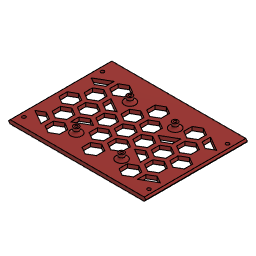
MCU Tray - BTT SKR Pico (Autodesk Fusion 360 design; units mm, degrees)
Autodesk Fusion 360 part; units mm, degrees
sketch "Sketch1" plane through (0, 0, 0) normal (0, 1, 0) x (1, 0, 0)
  line L0 (72.5, 2) -> (-72.5, 2)
  line L1 (-72.5, 2) -> (-72.5, -2) construction
  line L2 (-72.5, -2) -> (72.5, -2)
  line L3 (72.5, -2) -> (72.5, 2) construction
  line L4 (72.5, 2) -> (-72.5, -2) construction
  line L5 (-72.5, 2) -> (72.5, -2) construction
  line L6 (-72.5, 0) -> (-74.3, 0) construction
  line L7 (-72.5, -2) -> (-74.3, -0.2)
  line L8 (-74.3, 0.2) -> (-72.5, 2)
  line L9 (-74.3, -0.2) -> (-74.3, 0)
  line L10 (-74.3, 0) -> (-74.3, 0.2)
  line L11 (0, 0) -> (0, -2) construction
  line L12 (72.5, -2) -> (74.3, -0.2)
  line L13 (74.3, -0.2) -> (74.3, 0)
  line L14 (74.3, 0) -> (74.3, 0.2)
  line L15 (74.3, 0.2) -> (72.5, 2)
  dimension "d1" = 145
  dimension "d2" = 4
  dimension "d3" = 0.2
  constraint horizontal L0
  constraint perpendicular L0 L1
  constraint parallel L0 L2
  constraint parallel L1 L3
  constraint coincident L4 L11.start
  constraint coincident L5 L11.start
  constraint coincident L11.start origin
  constraint midpoint L1 L6.start
  constraint perpendicular L1 L6
  constraint coincident L5 L0.end
  constraint coincident L0 L1.start
  constraint perpendicular L6 L9
  constraint perpendicular L6 L10
  constraint midpoint L2 L11.end
  constraint symmetric L1.end L11 L2.end
  constraint symmetric L0.end L11 L0.start
  constraint symmetric L7.end L11 L12.end
  constraint symmetric L6.end L11 L13.end
  constraint symmetric L8.start L11 L14.end
  measures "d1" distance of L1.end L2.end
  measures "d2" distance of L0.end L1.end
  measures "d3" distance of L7.end L6.end
extrude "Extrude1" add sketch "Sketch1" along normal blind 190 and the other way blind 15
sketch "Sketch2" plane through (0, 0, 2) normal (0, 0, 1) x (-1, 0, 0)
  line L0 (72.5, 15) -> (-72.5, 15)
  line L1 (-72.5, 15) -> (-72.5, -190)
  line L2 (-72.5, -190) -> (72.5, -190)
  line L3 (72.5, -190) -> (72.5, 15)
  line L4 (0, 0) -> (0, -13.083) construction
  circle A0 centre (-67.6414, -9.9998) radius 2.3
  line L5 (72.6414, -59.8458) -> (72.6414, 0.0002) construction
  circle A1 centre (67.6414, -9.9998) radius 2.3
  line L6 (72.5, -190) -> (72.5, 15)
  line L7 (72.6414, 0.0002) -> (67.6414, 0.0002) construction
  line L8 (67.6414, 0.0002) -> (67.6414, -9.9998) construction
  line L9 (67.6414, -9.9998) -> (72.6414, -9.9998) construction
  line L10 (72.6414, -9.9998) -> (72.6414, 0.0002) construction
  line L11 (67.6414, -9.9998) -> (67.6414, -94.9998) construction
  circle A2 centre (67.6414, -94.9998) radius 2.3
  circle A3 centre (-67.6414, -94.9998) radius 2.3
  circle A4 centre (-67.6414, -9.9998) radius 1.8
  circle A5 centre (67.6414, -9.9998) radius 1.8
  circle A6 centre (67.6414, -94.9998) radius 1.8
  circle A7 centre (-67.6414, -94.9998) radius 1.8
  dimension "d14" = 5
  dimension "d15" = 10
  dimension "d16" = 4.6
  dimension "d17" = 85
  dimension "d18" = 4.6
  dimension "d59" = 3.6
  dimension "d60" = 3.6
  dimension "d61" = 3.6
  dimension "d62" = 3.6
  constraint coincident L4.start origin
  constraint vertical L4
  constraint symmetric L4 A0 A1
  constraint horizontal L7
  constraint vertical L8
  constraint horizontal L9
  constraint vertical L10
  constraint coincident A1.centre L8.end
  constraint perpendicular L9 L11
  constraint coincident L11.end A2.centre
  constraint symmetric L4 A2 A3
  constraint concentric A0 A4
  constraint concentric A1 A5
  constraint concentric A2 A6
  constraint concentric A3 A7
  measures "d14" distance of L5.end L7.end
  measures "d15" distance of L5.end L9.end
  measures "d16" diameter of A1
  measures "d17" distance of A1.centre L11.end
  measures "d18" diameter of A2
  measures "d59" diameter of A4
  measures "d60" diameter of A5
  measures "d61" diameter of A6
  measures "d62" diameter of A7
extrude "Extrude2" cut sketch "Sketch2" against normal up to surface (4 mm away) contours A0 | A1 | A2 | A3 | A4 | A5 | A6 | A7
extrude "Extrude3" cut 1 faces at (24.1667, 190, 0.6667) along direction (0, -1, 0) blind 40.154
extrude "Extrude10" add sketch "Sketch2" against normal blind 4 contours A0 | A1 | A2 | A3
sketch "Sketch3" plane through (0, 0, 2) normal (0, 0, 1) x (-1, 0, 0)
  line L0 (-72.5, -149.846) -> (72.5, -149.846)
  line L1 (72.5, -149.846) -> (72.5, 15)
  line L2 (72.5, 15) -> (-72.5, 15)
  line L3 (-72.5, 15) -> (-72.5, -149.846)
  line L4 (67.6414, -94.9998) -> (-67.6414, -9.9998) construction
  line L5 (-24.5, -23.4998) -> (24.5, -81.4998) construction
  line L6 (24.5, -23.4998) -> (-24.5, -81.4998) construction
  circle A0 centre (24.5, -81.4998) radius 2.35
  circle A1 centre (-24.5, -81.4998) radius 3
  circle A2 centre (24.5, -81.4998) radius 3
  circle A3 centre (-24.5, -81.4998) radius 2.35
  circle A4 centre (24.5, -23.4998) radius 2.35
  circle A5 centre (24.5, -23.4998) radius 3
  circle A6 centre (-24.5, -23.4998) radius 3
  circle A7 centre (-24.5, -23.4998) radius 2.35
  circle A8 centre (24.5, -23.4998) radius 1.4
  circle A9 centre (-24.5, -23.4998) radius 1.4
  circle A10 centre (-24.5, -81.4998) radius 1.4
  circle A11 centre (24.5, -81.4998) radius 1.4
  circle A12 centre (67.6414, -94.9998) radius 1.8
  circle A13 centre (-67.6414, -94.9998) radius 1.8
  circle A14 centre (67.6414, -9.9998) radius 1.8
  circle A15 centre (-67.6414, -9.9998) radius 1.8
  point P0 (0, -52.4998)
  dimension "d19" = 49
  dimension "d20" = 58
  dimension "d21" = 4.7
  dimension "d22" = 6
  dimension "d23" = 6
  dimension "d24" = 4.7
  dimension "d25" = 4.7
  dimension "d26" = 6
  dimension "d27" = 6
  dimension "d28" = 4.7
  dimension "d33" = 2.8
  dimension "d34" = 2.8
  dimension "d35" = 2.8
  dimension "d36" = 2.8
  constraint coincident L5 P0
  constraint coincident L6 P0
  constraint midpoint L4 P0
  constraint coincident L5.end A0.centre
  constraint coincident L6.end A1.centre
  constraint concentric A0 A2
  constraint concentric A1 A3
  constraint coincident L6.start A4.centre
  constraint concentric A4 A5
  constraint coincident L5.start A6.centre
  constraint concentric A6 A7
  constraint concentric A4 A8
  constraint concentric A6 A9
  constraint concentric A1 A10
  measures "d19" distance of L5.end L6.end
  measures "d20" distance of L6.start L5.end
  measures "d21" diameter of A0
  measures "d22" diameter of A1
  measures "d23" diameter of A2
  measures "d24" diameter of A3
  measures "d25" diameter of A4
  measures "d26" diameter of A5
  measures "d27" diameter of A6
  measures "d28" diameter of A7
  measures "d33" diameter of A8
  measures "d34" diameter of A9
  measures "d35" diameter of A10
  measures "d36" diameter of A11
extrude "Extrude4" cut sketch "Sketch3" against normal blind 4 contours A8 | A9 | A10 | A11
extrude "Extrude5" add sketch "Sketch3" along normal blind 6 contours A0 | A1 | A2 | A3 | A4 | A5 | A6 | A7
extrude "Extrude7" cut 1 faces at (24.1667, -15, 0.6667) along direction (0, 1, 0) blind 15
extrude "Extrude8" cut 1 faces at (24.1667, 149.846, 0.6667) along direction (0, -1, 0) blind 40
sketch "Sketch4" plane through (0, 0, 2) normal (0, 0, 1) x (-1, 0, 0)
  line L0 (-72.5, -109.846) -> (72.5, -109.846)
  line L1 (72.5, -109.846) -> (72.5, 0)
  line L2 (72.5, 0) -> (-72.5, 0)
  line L3 (-72.5, 0) -> (-72.5, -109.846)
  line L4 (-24.5, -23.4998) -> (24.5, -81.4998) construction
  line L5 (24.5, -81.4998) -> (24.5, -23.4998) construction
  line L6 (24.5, -23.4998) -> (-24.5, -81.4998) construction
  line L7 (0, -43.4998) -> (-7.7942, -47.9998)
  line L8 (-7.7942, -47.9998) -> (-7.7942, -56.9998)
  line L9 (-7.7942, -56.9998) -> (0, -61.4998)
  line L10 (0, -61.4998) -> (7.7942, -56.9998)
  line L11 (7.7942, -56.9998) -> (7.7942, -47.9998)
  line L12 (7.7942, -47.9998) -> (0, -43.4998)
  line L13 (52.2058, -47.9998) -> (52.2058, -56.9998)
  line L14 (52.2058, -56.9998) -> (60, -61.4998)
  line L15 (60, -61.4998) -> (67.7942, -56.9998)
  line L16 (67.7942, -56.9998) -> (67.7942, -47.9998)
  line L17 (67.7942, -47.9998) -> (60, -43.4998)
  line L18 (60, -43.4998) -> (52.2058, -47.9998)
  line L19 (32.2058, -47.9998) -> (32.2058, -56.9998)
  line L20 (32.2058, -56.9998) -> (40, -61.4998)
  line L21 (40, -61.4998) -> (47.7942, -56.9998)
  line L22 (47.7942, -56.9998) -> (47.7942, -47.9998)
  line L23 (47.7942, -47.9998) -> (40, -43.4998)
  line L24 (40, -43.4998) -> (32.2058, -47.9998)
  line L25 (12.2058, -47.9998) -> (12.2058, -56.9998)
  line L26 (12.2058, -56.9998) -> (20, -61.4998)
  line L27 (20, -61.4998) -> (27.7942, -56.9998)
  line L28 (27.7942, -56.9998) -> (27.7942, -47.9998)
  line L29 (27.7942, -47.9998) -> (20, -43.4998)
  line L30 (20, -43.4998) -> (12.2058, -47.9998)
  line L31 (-27.7942, -47.9998) -> (-27.7942, -56.9998)
  line L32 (-27.7942, -56.9998) -> (-20, -61.4998)
  line L33 (-20, -61.4998) -> (-12.2058, -56.9998)
  line L34 (-12.2058, -56.9998) -> (-12.2058, -47.9998)
  line L35 (-12.2058, -47.9998) -> (-20, -43.4998)
  line L36 (-20, -43.4998) -> (-27.7942, -47.9998)
  line L37 (-47.7942, -47.9998) -> (-47.7942, -56.9998)
  line L38 (-47.7942, -56.9998) -> (-40, -61.4998)
  line L39 (-40, -61.4998) -> (-32.2058, -56.9998)
  line L40 (-32.2058, -56.9998) -> (-32.2058, -47.9998)
  line L41 (-32.2058, -47.9998) -> (-40, -43.4998)
  line L42 (-40, -43.4998) -> (-47.7942, -47.9998)
  line L43 (10, -60.8203) -> (2.2058, -65.3203)
  line L44 (2.2058, -65.3203) -> (2.2058, -74.3203)
  line L45 (2.2058, -74.3203) -> (10, -78.8203)
  line L46 (10, -78.8203) -> (17.7942, -74.3203)
  line L47 (17.7942, -74.3203) -> (17.7942, -65.3203)
  line L48 (17.7942, -65.3203) -> (10, -60.8203)
  line L49 (77.7942, -65.3203) -> (70, -60.8203) construction
  line L50 (70, -60.8203) -> (62.2058, -65.3203) construction
  line L51 (62.2058, -65.3203) -> (62.2058, -74.3203) construction
  line L52 (62.2058, -74.3203) -> (70, -78.8203) construction
  line L53 (77.7942, -74.3203) -> (77.7942, -65.3203) construction
  line L54 (70, -78.8203) -> (77.7942, -74.3203) construction
  line L55 (57.7942, -65.3203) -> (50, -60.8203)
  line L56 (50, -60.8203) -> (42.2058, -65.3203)
  line L57 (42.2058, -65.3203) -> (42.2058, -74.3203)
  line L58 (42.2058, -74.3203) -> (50, -78.8203)
  line L59 (57.7942, -74.3203) -> (57.7942, -65.3203)
  line L60 (50, -78.8203) -> (57.7942, -74.3203)
  line L61 (37.7942, -65.3203) -> (30, -60.8203)
  line L62 (30, -60.8203) -> (22.2058, -65.3203)
  line L63 (22.2058, -65.3203) -> (22.2058, -74.3203) construction
  line L64 (22.2058, -74.3203) -> (30, -78.8203) construction
  line L65 (37.7942, -74.3203) -> (37.7942, -65.3203)
  line L66 (30, -78.8203) -> (37.7942, -74.3203) construction
  line L67 (-2.2058, -65.3203) -> (-10, -60.8203)
  line L68 (-10, -60.8203) -> (-17.7942, -65.3203)
  line L69 (-17.7942, -65.3203) -> (-17.7942, -74.3203)
  line L70 (-17.7942, -74.3203) -> (-10, -78.8203)
  line L71 (-2.2058, -74.3203) -> (-2.2058, -65.3203)
  line L72 (-10, -78.8203) -> (-2.2058, -74.3203)
  line L73 (-22.2058, -65.3203) -> (-30, -60.8203)
  line L74 (-30, -60.8203) -> (-37.7942, -65.3203)
  line L75 (-37.7942, -65.3203) -> (-37.7942, -74.3203)
  line L76 (-37.7942, -74.3203) -> (-30, -78.8203) construction
  line L77 (-22.2058, -74.3203) -> (-22.2058, -65.3203) construction
  line L78 (-30, -78.8203) -> (-22.2058, -74.3203) construction
  line L79 (-67.7942, -47.9998) -> (-67.7942, -56.9998)
  line L80 (-67.7942, -56.9998) -> (-60, -61.4998)
  line L81 (-60, -61.4998) -> (-52.2058, -56.9998)
  line L82 (-52.2058, -56.9998) -> (-52.2058, -47.9998)
  line L83 (-52.2058, -47.9998) -> (-60, -43.4998)
  line L84 (-60, -43.4998) -> (-67.7942, -47.9998)
  line L85 (-42.2058, -65.3203) -> (-50, -60.8203)
  line L86 (-50, -60.8203) -> (-57.7942, -65.3203)
  line L87 (-57.7942, -65.3203) -> (-57.7942, -74.3203)
  line L88 (-57.7942, -74.3203) -> (-50, -78.8203)
  line L89 (-42.2058, -74.3203) -> (-42.2058, -65.3203)
  line L90 (-50, -78.8203) -> (-42.2058, -74.3203)
  line L91 (2.2058, -39.6793) -> (10, -44.1793)
  line L92 (10, -44.1793) -> (17.7942, -39.6793)
  line L93 (17.7942, -39.6793) -> (17.7942, -30.6793)
  line L94 (17.7942, -30.6793) -> (10, -26.1793)
  line L95 (10, -26.1793) -> (2.2058, -30.6793)
  line L96 (2.2058, -30.6793) -> (2.2058, -39.6793)
  line L97 (77.7942, -39.6793) -> (77.7942, -30.6793) construction
  line L98 (77.7942, -30.6793) -> (70, -26.1793) construction
  line L99 (70, -26.1793) -> (62.2058, -30.6793) construction
  line L100 (62.2058, -30.6793) -> (62.2058, -39.6793) construction
  line L101 (70, -44.1793) -> (77.7942, -39.6793) construction
  line L102 (62.2058, -39.6793) -> (70, -44.1793) construction
  line L103 (57.7942, -39.6793) -> (57.7942, -30.6793)
  line L104 (57.7942, -30.6793) -> (50, -26.1793)
  line L105 (50, -26.1793) -> (42.2058, -30.6793)
  line L106 (42.2058, -30.6793) -> (42.2058, -39.6793)
  line L107 (50, -44.1793) -> (57.7942, -39.6793)
  line L108 (42.2058, -39.6793) -> (50, -44.1793)
  line L109 (37.7942, -39.6793) -> (37.7942, -30.6793)
  line L110 (37.7942, -30.6793) -> (30, -26.1793) construction
  line L111 (30, -26.1793) -> (22.2058, -30.6793) construction
  line L112 (22.2058, -30.6793) -> (22.2058, -39.6793) construction
  line L113 (30, -44.1793) -> (37.7942, -39.6793)
  line L114 (22.2058, -39.6793) -> (30, -44.1793)
  line L115 (-2.2058, -39.6793) -> (-2.2058, -30.6793)
  line L116 (-2.2058, -30.6793) -> (-10, -26.1793)
  line L117 (-10, -26.1793) -> (-17.7942, -30.6793)
  line L118 (-17.7942, -30.6793) -> (-17.7942, -39.6793)
  line L119 (-10, -44.1793) -> (-2.2058, -39.6793)
  line L120 (-17.7942, -39.6793) -> (-10, -44.1793)
  line L121 (-22.2058, -39.6793) -> (-22.2058, -30.6793) construction
  line L122 (-22.2058, -30.6793) -> (-30, -26.1793) construction
  line L123 (-30, -26.1793) -> (-37.7942, -30.6793) construction
  line L124 (-37.7942, -30.6793) -> (-37.7942, -39.6793)
  line L125 (-30, -44.1793) -> (-22.2058, -39.6793)
  line L126 (-37.7942, -39.6793) -> (-30, -44.1793)
  line L127 (-42.2058, -39.6793) -> (-42.2058, -30.6793)
  line L128 (-42.2058, -30.6793) -> (-50, -26.1793)
  line L129 (-50, -26.1793) -> (-57.7942, -30.6793)
  line L130 (-57.7942, -30.6793) -> (-57.7942, -39.6793)
  line L131 (-50, -44.1793) -> (-42.2058, -39.6793)
  line L132 (-57.7942, -39.6793) -> (-50, -44.1793)
  line L133 (-87.7942, -47.9998) -> (-87.7942, -56.9998) construction
  line L134 (-87.7942, -56.9998) -> (-80, -61.4998) construction
  line L135 (-80, -61.4998) -> (-72.2058, -56.9998) construction
  line L136 (-72.2058, -56.9998) -> (-72.2058, -47.9998) construction
  line L137 (-72.2058, -47.9998) -> (-80, -43.4998) construction
  line L138 (-80, -43.4998) -> (-87.7942, -47.9998) construction
  line L139 (-62.2058, -65.3203) -> (-70, -60.8203) construction
  line L140 (-70, -60.8203) -> (-77.7942, -65.3203) construction
  line L141 (-77.7942, -65.3203) -> (-77.7942, -74.3203) construction
  line L142 (-77.7942, -74.3203) -> (-70, -78.8203) construction
  line L143 (-62.2058, -74.3203) -> (-62.2058, -65.3203) construction
  line L144 (-70, -78.8203) -> (-62.2058, -74.3203) construction
  line L145 (-62.2058, -39.6793) -> (-62.2058, -30.6793) construction
  line L146 (-62.2058, -30.6793) -> (-70, -26.1793) construction
  line L147 (-70, -26.1793) -> (-77.7942, -30.6793) construction
  line L148 (-77.7942, -30.6793) -> (-77.7942, -39.6793) construction
  line L149 (-70, -44.1793) -> (-62.2058, -39.6793) construction
  line L150 (-77.7942, -39.6793) -> (-70, -44.1793) construction
  line L151 (-67.7942, -82.9998) -> (-67.7942, -91.9998) construction
  line L152 (-67.7942, -91.9998) -> (-60, -96.4998) construction
  line L153 (-60, -96.4998) -> (-52.2058, -91.9998) construction
  line L154 (-52.2058, -91.9998) -> (-52.2058, -82.9998)
  line L155 (-52.2058, -82.9998) -> (-60, -78.4998)
  line L156 (-60, -78.4998) -> (-67.7942, -82.9998)
  line L157 (-47.7942, -91.9998) -> (-40, -96.4998)
  line L158 (-40, -96.4998) -> (-32.2058, -91.9998)
  line L159 (-32.2058, -91.9998) -> (-32.2058, -82.9998)
  line L160 (-32.2058, -82.9998) -> (-40, -78.4998)
  line L161 (-47.7942, -82.9998) -> (-47.7942, -91.9998)
  line L162 (-40, -78.4998) -> (-47.7942, -82.9998)
  line L163 (-27.7942, -91.9998) -> (-20, -96.4998)
  line L164 (-20, -96.4998) -> (-12.2058, -91.9998)
  line L165 (-12.2058, -91.9998) -> (-12.2058, -82.9998)
  line L166 (-12.2058, -82.9998) -> (-20, -78.4998)
  line L167 (-27.7942, -82.9998) -> (-27.7942, -91.9998)
  line L168 (-20, -78.4998) -> (-27.7942, -82.9998)
  line L169 (-7.7942, -91.9998) -> (0, -96.4998)
  line L170 (0, -96.4998) -> (7.7942, -91.9998)
  line L171 (7.7942, -91.9998) -> (7.7942, -82.9998)
  line L172 (7.7942, -82.9998) -> (0, -78.4998)
  line L173 (-7.7942, -82.9998) -> (-7.7942, -91.9998)
  line L174 (0, -78.4998) -> (-7.7942, -82.9998)
  line L175 (12.2058, -91.9998) -> (20, -96.4998)
  line L176 (20, -96.4998) -> (27.7942, -91.9998)
  line L177 (27.7942, -91.9998) -> (27.7942, -82.9998)
  line L178 (27.7942, -82.9998) -> (20, -78.4998)
  line L179 (12.2058, -82.9998) -> (12.2058, -91.9998)
  line L180 (20, -78.4998) -> (12.2058, -82.9998)
  line L181 (32.2058, -91.9998) -> (40, -96.4998)
  line L182 (40, -96.4998) -> (47.7942, -91.9998)
  line L183 (47.7942, -91.9998) -> (47.7942, -82.9998)
  line L184 (47.7942, -82.9998) -> (40, -78.4998)
  line L185 (32.2058, -82.9998) -> (32.2058, -91.9998)
  line L186 (40, -78.4998) -> (32.2058, -82.9998)
  line L187 (52.2058, -91.9998) -> (60, -96.4998) construction
  line L188 (60, -96.4998) -> (67.7942, -91.9998) construction
  line L189 (67.7942, -91.9998) -> (67.7942, -82.9998) construction
  line L190 (67.7942, -82.9998) -> (60, -78.4998)
  line L191 (52.2058, -82.9998) -> (52.2058, -91.9998)
  line L192 (60, -78.4998) -> (52.2058, -82.9998)
  line L193 (-67.7942, -12.9998) -> (-67.7942, -21.9998) construction
  line L194 (-67.7942, -21.9998) -> (-60, -26.4998)
  line L195 (-60, -26.4998) -> (-52.2058, -21.9998)
  line L196 (-52.2058, -21.9998) -> (-52.2058, -12.9998)
  line L197 (-52.2058, -12.9998) -> (-60, -8.4998) construction
  line L198 (-60, -8.4998) -> (-67.7942, -12.9998) construction
  line L199 (-47.7942, -21.9998) -> (-40, -26.4998)
  line L200 (-40, -26.4998) -> (-32.2058, -21.9998)
  line L201 (-32.2058, -21.9998) -> (-32.2058, -12.9998)
  line L202 (-32.2058, -12.9998) -> (-40, -8.4998)
  line L203 (-47.7942, -12.9998) -> (-47.7942, -21.9998)
  line L204 (-40, -8.4998) -> (-47.7942, -12.9998)
  line L205 (-27.7942, -21.9998) -> (-20, -26.4998)
  line L206 (-20, -26.4998) -> (-12.2058, -21.9998)
  line L207 (-12.2058, -21.9998) -> (-12.2058, -12.9998)
  line L208 (-12.2058, -12.9998) -> (-20, -8.4998)
  line L209 (-27.7942, -12.9998) -> (-27.7942, -21.9998)
  line L210 (-20, -8.4998) -> (-27.7942, -12.9998)
  line L211 (-7.7942, -21.9998) -> (0, -26.4998)
  line L212 (0, -26.4998) -> (7.7942, -21.9998)
  line L213 (7.7942, -21.9998) -> (7.7942, -12.9998)
  line L214 (7.7942, -12.9998) -> (0, -8.4998)
  line L215 (-7.7942, -12.9998) -> (-7.7942, -21.9998)
  line L216 (0, -8.4998) -> (-7.7942, -12.9998)
  line L217 (12.2058, -21.9998) -> (20, -26.4998)
  line L218 (20, -26.4998) -> (27.7942, -21.9998)
  line L219 (27.7942, -21.9998) -> (27.7942, -12.9998)
  line L220 (27.7942, -12.9998) -> (20, -8.4998)
  line L221 (12.2058, -12.9998) -> (12.2058, -21.9998)
  line L222 (20, -8.4998) -> (12.2058, -12.9998)
  line L223 (32.2058, -21.9998) -> (40, -26.4998)
  line L224 (40, -26.4998) -> (47.7942, -21.9998)
  line L225 (47.7942, -21.9998) -> (47.7942, -12.9998)
  line L226 (47.7942, -12.9998) -> (40, -8.4998)
  line L227 (32.2058, -12.9998) -> (32.2058, -21.9998)
  line L228 (40, -8.4998) -> (32.2058, -12.9998)
  line L229 (52.2058, -21.9998) -> (60, -26.4998)
  line L230 (60, -26.4998) -> (67.7942, -21.9998)
  line L231 (67.7942, -21.9998) -> (67.7942, -12.9998) construction
  line L232 (67.7942, -12.9998) -> (60, -8.4998) construction
  line L233 (52.2058, -12.9998) -> (52.2058, -21.9998)
  line L234 (60, -8.4998) -> (52.2058, -12.9998) construction
  line L235 (67.7942, -82.9998) -> (52.2058, -91.9998)
  line L236 (52.2058, -12.9998) -> (67.7942, -21.9998)
  line L237 (-52.2058, -12.9998) -> (-67.7942, -21.9998)
  line L238 (-67.7942, -82.9998) -> (-52.2058, -91.9998)
  line L239 (-37.7942, -30.6793) -> (-22.2058, -39.6793)
  line L240 (-37.7942, -74.3203) -> (-22.2058, -65.3203)
  line L241 (37.7942, -74.3203) -> (22.2058, -65.3203)
  line L242 (22.2058, -39.6793) -> (37.7942, -30.6793)
  circle A0 centre (67.6414, -94.9998) radius 1.8
  circle A1 centre (-67.6414, -94.9998) radius 1.8
  circle A2 centre (67.6414, -9.9998) radius 1.8
  circle A3 centre (-67.6414, -9.9998) radius 1.8
  circle A4 centre (-24.5, -23.4998) radius 3
  circle A5 centre (24.5, -23.4998) radius 3
  circle A6 centre (24.5, -81.4998) radius 3
  circle A7 centre (-24.5, -81.4998) radius 3
  point P0 (0, -52.4998)
  dimension "d46" = 9
  dimension "d49" = -20
  dimension "d50" = 0
  dimension "d52" = 120
  dimension "d55" = 0
  dimension "d56" = 35
  constraint vertical L8
  constraint midpoint L6 P0
  measures "d46" distance of L7.start P0
extrude "Extrude9" cut sketch "Sketch4" against normal blind 4 contours L7 L8 L9 L10 L11 L12 | L13 L14 L15 L16 L17 L18 | L19 L20 L21 L22 L23 L24 | L25 L26 L27 L28 L29 L30 | L31 L32 L33 L34 L35 L36 | L37 L38 L39 L40 L41 L42 | L43 L44 L45 L46 L47 L48 | L55 L56 L57 L58 L59 L60 | L61 L62 L65 L241 | L67 L68 L69 L70 L71 L72 | L73 L74 L75 L240 | L79 L80 L81 L82 L83 L84 | L85 L86 L87 L88 L89 L90 | L91 L92 L93 L94 L95 L96 | L103 L104 L105 L106 L107 L108 | L109 L113 L114 L242 | L115 L116 L117 L118 L119 L120 | L124 L125 L126 L239 | L127 L128 L129 L130 L131 L132 | L154 L155 L156 L238 | L157 L158 L159 L160 L161 L162 | L169 L170 L171 L172 L173 L174 | L181 L182 L183 L184 L185 L186 | L190 L191 L192 L235 | L194 L195 L196 L237 | L199 L200 L201 L202 L203 L204 | L211 L212 L213 L214 L215 L216 | L223 L224 L225 L226 L227 L228 | L229 L230 L233 L236
fillet "Fillet1" radius 3 4 edges at (27.297, 22.415, 2) (-21.703, 22.415, 2) (-21.703, 80.415, 2) (27.297, 80.415, 2)
equation "d18 = d16"
equation "d21 = d25"
equation "d22 = d23"
equation "d23 = d26"
equation "d24 = d21"
equation "d27 = d26"
equation "d28 = d25"
equation "d33 = d36"
equation "d34 = d36"
equation "d35 = d36"
